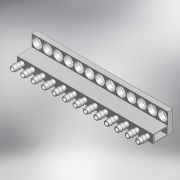
# Autodesk Inventor part: ManifoldExtension2
Saved by Autodesk Inventor 2018 (Build 220112000, 112)
## iProperties
Created: 2018-10-08
Part Number: ManifoldExtension2
Material: ABS Plastic
Document SubType Name: Modeling
Designer: Isaac Newcomb
Density: 1.06 g/cm^3
Appearance: Smooth - White
Width: 15.000 mm
FittingLength: 10.000 mm
Author: Isaac Newcomb
Autodesk Inventor part; units mm, degrees
ref_plane "YZ Plane" through (0, 0, 0) normal (1, 0, 0) x (0, 1, 0)
ref_plane "Silicone Fitting Plane" through (0, 0, -5.25) normal (0, 0, 1) x (1, 0, 0)
ref_plane "Cap Plane" through (0, 0, -136.5) normal (0, 0, 1) x (1, 0, 0)
sketch "Base Sketch" plane through (0, 0, 0) normal (0, 0, 1) x (1, 0, 0)
  line L0 (0, 0) -> (15, 0)
  line L1 (15, 0) -> (15, 8.1625)
  line L2 (15, 8.1625) -> (0, 8.1625)
  line L3 (0, 8.1625) -> (0, 0)
  line L4 (1.5, 1.5) -> (12, 1.5)
  line L5 (12, 1.5) -> (12, 6.6625)
  line L6 (12, 6.6625) -> (1.5, 6.6625)
  line L7 (1.5, 6.6625) -> (1.5, 1.5)
  line L8 (13.5, 0.75) -> (0.75, 0.75)
  line L9 (0.75, 0.75) -> (0.75, 7.4125)
  line L10 (0.75, 7.4125) -> (13.5, 7.4125)
  line L11 (13.5, 7.4125) -> (13.5, 0.75)
  dimension "Height" = 8.1625
  dimension "Width" = 15
  dimension "d1" = 1.5
  dimension "d2" = 1.5
  dimension "d3" = 1.5
  dimension "FittingWallWallThickness" = 3
  dimension "d181" = 0.75
  dimension "d182" = 0.75
  dimension "d183" = 1.5
  dimension "d184" = 0.75
  constraints: 24 end point, 6 parallel, 3 horizontal, 3 perpendicular
  measures "Height" distance of L2.end L0.start
  measures "Width" distance of L0.start L0.end
  measures "d1" distance between parallel lines of L3 L7
  measures "d2" distance between parallel lines of L2 L6
  measures "d3" distance between parallel lines of L4 L0
  measures "FittingWallWallThickness" distance between parallel lines of L1 L5
  measures "d181" distance between parallel lines of L8 L4
  measures "d182" distance between parallel lines of L6 L10
  measures "d183" distance between parallel lines of L5 L11
  measures "d184" distance between parallel lines of L7 L9
extrude "Base" add sketch "Base Sketch" against normal blind 136.5 contours L3 L2 L1 L0 | L8 L9 L10 L11
sketch "Sketch22" plane through (0, 0, 0) normal (0, 1, 0) x (-1, 0, 0)
  line L0 (5, -136.5) -> (0, -136.5)
  line L1 (0, -136.5) -> (0, 0)
  line L2 (0, 0) -> (5, 0)
  line L3 (5, 0) -> (5, -136.5)
  dimension "d161" = 136.5
  dimension "d162" = 5
  constraints: 8 end point, 2 parallel, 1 coincident, 1 horizontal, 1 perpendicular
  measures "d161" distance of L2.end L0.start
  measures "d162" distance of L0.start L0.end
extrude "Extrusion21" add sketch "Sketch22" along normal blind 8.1625 and the other way blind 12
sketch "Silicone Fitting Sketch" plane through (0, 0, -5.25) normal (0, 0, 1) x (1, 0, 0)
  line L0 (15, 4.0812) -> (25, 4.0812) construction
  line L1 (25, 4.0812) -> (25, 1.7)
  line L2 (25, 1.7) -> (22, 1)
  line L3 (22, 1) -> (22, 1.7)
  line L4 (22, 1.7) -> (19, 1)
  line L5 (19, 1) -> (19, 1.7)
  line L6 (19, 1.7) -> (15, 1.7)
  line L7 (15, 1.7) -> (15, 4.0812)
  line L8 (25, 1.7) -> (19, 1.7) construction
  line L9 (15, 2.2) -> (25, 2.2)
  line L10 (-5, 0) -> (30, 0) construction
  point P0 (0, 0)
  dimension "d184" = 0.75
  dimension "FittingLength" = 10
  dimension "FittingRadius" = 2.3813
  dimension "d4" = 0.5
  dimension "BarbHeight" = 0.7
  dimension "BarbLength" = 3
  dimension "d5" = 15
  dimension "FittingClearance" = 1
  constraints: 20 end point, 4 perpendicular, 3 parallel, 2 point on line, 1 collinear, 1 horizontal, 1 midpoint
  measures "FittingLength" distance of L0.start L0.end
  measures "FittingRadius" distance of L6.end L0.start
  measures "d4" distance between parallel lines of L6 L9
  measures "BarbHeight" distance of L2.end L3.end
  measures "BarbLength" horizontal distance of L3.end L4.end
  measures "d5" distance from line of point (0, 0) L7
  measures "FittingClearance" distance from line of L10 L4.end
revolve "Silicone Fitting" add sketch "Silicone Fitting Sketch" angle 360 about axis through (15, 4.0812, -5.25) along (1, 0, 0)
sketch "Airflow Cut Sketch" plane through (15, 4.0812, -5.25) normal (1, 0, 0) x (0, 0, -1)
  circle A0 centre (0, 0) radius 1.8812 projected
  point P0 (-5.25, -4.0812)
extrude "Airflow Cut" cut sketch "Airflow Cut Sketch" against normal blind 3
pattern_linear "Airflow Cut Repetition" count 13 spacing 10.5 along (0, 0, -1) of "Airflow Cut"
pattern_linear "Rectangular Pattern7" count 13 spacing 10.5 along (0, 0, -1) of "Silicone Fitting"
sketch "Sketch23" plane through (0, 0, 0) normal (1, 0, 0) x (0, 1, 0)
  circle A0 centre (-6, -5.25) radius 5
  point P0 (0, 0)
  dimension "d167" = 10
  dimension "d168" = 5.25
  dimension "d169" = 6
  constraints: 1 centre point
  measures "d167" diameter of A0
  measures "d168" vertical distance of A0.centre point (0, 0)
  measures "d169" horizontal distance of A0.centre point (0, 0)
extrude "Extrusion22" cut sketch "Sketch23" against normal through all
pattern_linear "Rectangular Pattern8" count 13 spacing 10.5 along (0, 0, -1) of "Extrusion22"
extrude "Extrusion24" cut sketch "Base Sketch" against normal blind 10.5 contours L8 L9 L10 L11
equation "\"Height\" = 2 * FittingRadius + 2 * FittingClearance + 2 * BarbHeight"
equation "\"Width\" = ManifoldWidth"
equation "\"d1\" = WallThickness"
equation "\"d2\" = WallThickness"
equation "\"d3\" = WallThickness"
equation "\"FittingWallWallThickness\" = 2 * WallThickness"
equation "\"d161\" = Length"
equation "\"d163\" = Height"
equation "\"FittingLength\" = ManifoldFittingLength"
equation "\"d5\" = Width"
equation "\"d112\" = FittingWallWallThickness"
equation "\"d157\" = KeyWidth + KeySpacing"
equation "\"d160\" = KeyWidth + KeySpacing"
equation "\"d167\" = KeyWidth"
equation "\"d168\" = 0.5 * KeySpacing + 0.5 * KeyWidth"
equation "\"d169\" = 0.5 * KeyWidth + 2 * KeySpacing"
equation "\"d174\" = KeyWidth + KeySpacing"
equation "\"WallThickness\" = 1.5"
equation "\"ManifoldWidth\" = 15"
equation "\"Length\" = 136.5"
equation "\"ManifoldFittingLength\" = 10"
equation "\"KeyWidth\" = 10"
equation "\"KeySpacing\" = 0.5"
body "Solid3"
